Autodesk Fusion 360 part; units mm, degrees
(part 3 of 3)
  line L460 (365.2476, 258.4329) -> (365.2434, 258.3962)
  line L461 (365.4242, 258.127) -> (365.9464, 257.9803)
  line L462 (368.5391, 247.253) -> (369.0636, 246.6115)
  line L463 (368.5276, 247.6061) -> (368.8896, 247.9996)
  arc A277 (389.0677, 270.0365) -> (388.9102, 270.1312) centre (381.1421, 257.037) ccw
  line L464 (390.9137, 269.3965) -> (390.4979, 269.0483)
  line L465 (368.5391, 247.253) -> (368.5181, 247.2786)
  line L466 (359.931, 254.736) -> (359.9373, 254.7725)
  arc A278 (365.4068, 257.7213) -> (365.1921, 257.4738) centre (365.4421, 257.4738) ccw
  line L467 (386.2134, 242.1256) -> (385.951, 242.5914)
  line L468 (386.5528, 242.0274) -> (386.5219, 242.0153)
  line L469 (337.8939, 271.7181) -> (337.924, 271.7319)
  arc A279 (389.0905, 270.6345) -> (388.9718, 270.9399) centre (388.8551, 270.7188) ccw
  line L470 (365.9769, 261.9967) -> (365.9644, 261.9618)
  line L471 (365.6981, 261.0428) -> (365.5104, 260.2357)
  arc A280 (391.238, 269.3938) -> (390.9137, 269.3965) centre (391.0742, 269.2049) ccw
  line L472 (365.6509, 259.9116) -> (366.1529, 259.7063)
  line L473 (390.5886, 269.6398) -> (390.3522, 269.1604)
  line L474 (349.1921, 271.9615) -> (349.0339, 271.6922)
  line L475 (345.0126, 272.9687) -> (344.1728, 272.9927)
  line L476 (386.1921, 271.9615) -> (385.9174, 271.4938)
  line L477 (347.7954, 241.5055) -> (347.7633, 241.4971)
  line L478 (348.8153, 272.0785) -> (348.78, 271.7745)
  line L479 (383.0125, 241.1919) -> (383.8327, 241.3099)
  line L480 (382.3002, 241.324) -> (382.3711, 241.8617)
  line L481 (384.4579, 272.4399) -> (384.2384, 271.9439)
  line L482 (365.972, 252.7816) -> (366.5131, 252.8189)
  line L483 (365.5152, 253.8176) -> (365.5077, 253.8498)
  line L484 (367.9424, 265.9998) -> (367.4944, 265.3027)
  line L485 (347.7954, 241.5055) -> (348.608, 241.7191)
  line L486 (384.7859, 272.5711) -> (384.75, 272.5805)
  line L487 (339.6082, 272.3347) -> (339.6397, 272.3449)
  line L488 (367.5178, 264.9502) -> (367.9217, 264.5882)
  line L489 (382.0224, 241.1057) -> (382.0595, 241.1067)
  line L490 (349.2026, 242.1214) -> (349.0524, 242.3881)
  line L491 (383.0125, 241.1919) -> (382.9797, 241.1872)
  line L492 (345.0224, 241.1057) -> (345.0595, 241.1067)
  line L493 (349.5329, 272.0545) -> (349.4983, 272.0679)
  line L494 (339.9414, 272.2172) -> (340.0761, 271.9424)
  line L495 (345.3002, 241.324) -> (345.341, 241.6336)
  line L496 (367.3232, 264.5938) -> (367.8315, 264.428)
  line L497 (383.8116, 272.7672) -> (383.8444, 272.7625)
  line L498 (381.1941, 241.082) -> (382.0224, 241.1057)
  line L499 (347.7859, 272.5711) -> (347.75, 272.5805)
  line L500 (346.823, 272.7656) -> (345.9914, 272.8852)
  line L501 (341.3815, 272.7518) -> (340.5581, 272.5849)
  line L502 (346.0011, 241.1903) -> (345.9683, 241.1856)
  line L503 (367.0067, 264.4367) -> (367.0213, 264.4665)
  line L504 (381.1941, 241.082) -> (381.161, 241.0811)
  line L505 (367.0067, 264.4367) -> (366.6411, 263.6931)
  line L506 (341.6992, 272.5971) -> (341.8017, 272.3087)
  line L507 (367.9424, 265.9998) -> (367.9603, 266.0277)
  line L508 (365.7029, 253.0104) -> (365.7113, 252.9744)
  line L509 (384.0588, 272.5148) -> (384.0582, 271.9802)
  line L510 (366.092, 252.3937) -> (366.5651, 252.6426)
  line L511 (350.3158, 271.7496) -> (349.5329, 272.0545)
  line L512 (383.8116, 272.7672) -> (382.9914, 272.8852)
  line L513 (342.3537, 272.8921) -> (342.3169, 272.889)
  line L514 (365.6608, 254.1395) -> (366.1592, 254.3329)
  line L515 (340.3216, 272.3225) -> (340.3342, 272.0104)
  line L516 (365.9841, 252.0572) -> (366.2625, 251.2767)
  line L517 (346.0011, 241.1903) -> (346.8327, 241.3099)
  line L518 (382.9914, 272.8852) -> (382.9547, 272.8904)
  line L519 (367.4944, 265.3027) -> (367.4743, 265.2716)
  line L520 (380.9075, 241.2886) -> (380.8169, 241.8155)
  line L521 (340.5581, 272.5849) -> (340.5218, 272.5776)
  line L522 (365.5858, 254.5386) -> (366.1276, 254.514)
  line L523 (365.5152, 253.8176) -> (365.7029, 253.0104)
  line L524 (382.7042, 241.3645) -> (382.5542, 241.8777)
  line L525 (343.1909, 272.964) -> (342.3537, 272.8921)
  line L526 (383.8327, 241.3099) -> (383.8694, 241.3151)
  line L527 (345.287, 272.746) -> (345.3215, 272.4419)
  line L528 (385.8041, 272.0814) -> (385.7425, 271.5504)
  line L529 (365.9841, 252.0572) -> (365.9729, 252.0884)
  line L530 (385.5873, 272.3604) -> (384.7859, 272.5711)
  line L531 (384.0838, 241.5584) -> (384.0929, 242.1007)
  line L532 (368.5086, 266.4517) -> (368.8686, 266.046)
  line L533 (345.9914, 272.8852) -> (345.9547, 272.8904)
  line L534 (368.2747, 266.1198) -> (368.7607, 265.8972)
  line L535 (385.5873, 272.3604) -> (385.6193, 272.352)
  line L536 (344.1728, 272.9927) -> (344.1357, 272.9937)
  line L537 (348.829, 241.9946) -> (348.7987, 242.3055)
  arc A281 (388.1768, 271.3594) -> (387.8604, 271.2886) centre (388.0602, 271.1382) ccw
  arc A282 (369.3939, 267.5274) -> (369.071, 267.4717) centre (369.2646, 267.3134) ccw
  arc A283 (367.1471, 263.0319) -> (367.0757, 262.8626) centre (381.1421, 257.037) ccw
  arc A284 (382.9547, 272.8904) -> (382.6805, 272.7174) centre (382.9191, 272.643) ccw
  arc A285 (353.6743, 269.196) -> (353.4628, 269.3589) centre (344.1421, 257.037) ccw
  arc A286 (365.1921, 256.575) -> (365.4024, 256.3282) centre (365.4421, 256.575) ccw
  arc A287 (353.5982, 269.6333) -> (353.515, 269.9503) centre (353.3739, 269.7439) ccw
  arc A288 (367.4743, 265.2716) -> (367.5178, 264.9502) centre (367.6846, 265.1364) ccw
  line L538 (380.2007, 241.1092) -> (380.2376, 241.106)
  arc A289 (365.7113, 252.9744) -> (365.972, 252.7816) centre (365.9548, 253.031) ccw
  line L539 (380.4773, 272.7732) -> (380.5978, 272.2523)
  arc A290 (352.4494, 243.6553) -> (352.7749, 243.6177) centre (352.6338, 243.8241) ccw
  arc A291 (350.3595, 242.3414) -> (350.5132, 242.6269) centre (350.2688, 242.5744) ccw
  line L540 (366.7045, 263.3456) -> (367.1471, 263.0319)
  line L541 (381.1728, 272.9927) -> (381.1357, 272.9937)
  arc A292 (368.2747, 266.1198) -> (367.9603, 266.0277) centre (368.1706, 265.8925) ccw
  arc A293 (386.4983, 272.0679) -> (386.1921, 271.9615) centre (386.4076, 271.8349) ccw
  arc A294 (368.5021, 266.7759) -> (368.5086, 266.4517) centre (368.6956, 266.6176) ccw
  line L542 (382.2754, 272.7464) -> (382.3358, 272.2152)
  line L543 (366.5519, 262.9693) -> (367.0757, 262.8626)
  arc A295 (365.6608, 254.1395) -> (365.5077, 253.8498) centre (365.7512, 253.9064) ccw
  line L544 (382.6805, 272.7174) -> (382.5189, 272.1997)
  arc A296 (385.8041, 272.0814) -> (385.6193, 272.352) centre (385.5558, 272.1102) ccw
  arc A297 (367.9217, 264.5882) -> (367.8315, 264.428) centre (381.1421, 257.037) ccw
  arc A298 (369.9756, 267.3863) -> (369.8514, 267.2508) centre (381.1421, 257.037) ccw
  line L545 (366.2554, 262.7772) -> (366.2665, 262.8084)
  arc A299 (352.1007, 270.6291) -> (351.982, 270.9345) centre (351.8653, 270.7134) ccw
  arc A300 (366.5519, 262.9693) -> (366.2665, 262.8084) centre (366.5019, 262.7244) ccw
  line L546 (382.0011, 272.969) -> (382.0342, 272.968)
  arc A301 (384.0588, 272.5148) -> (383.8444, 272.7625) centre (383.8088, 272.5151) ccw
  line L547 (382.0011, 272.969) -> (381.1728, 272.9927)
  line L548 (345.6928, 241.3629) -> (345.6069, 241.6566)
  arc A302 (384.75, 272.5805) -> (384.4579, 272.4399) centre (384.6865, 272.3387) ccw
  arc A303 (382.2754, 272.7464) -> (382.0342, 272.968) centre (382.027, 272.7182) ccw
  arc A304 (350.8699, 242.7955) -> (351.189, 242.7211) centre (351.0723, 242.9422) ccw
  arc A305 (352.0143, 243.743) -> (352.2428, 243.881) centre (344.1421, 257.037) ccw
  arc A306 (365.3488, 254.7598) -> (365.5858, 254.5386) centre (365.5971, 254.7883) ccw
  arc A307 (366.092, 252.3937) -> (365.9729, 252.0884) centre (366.2084, 252.1724) ccw
  arc A308 (365.4314, 255.9231) -> (365.2463, 255.6528) centre (365.4947, 255.6813) ccw
  arc A309 (350.4476, 242.9323) -> (350.6903, 243.0433) centre (344.1421, 257.037) ccw
  arc A310 (381.1357, 272.9937) -> (380.883, 272.7906) centre (381.1286, 272.7438) ccw
  arc A311 (336.6123, 270.8712) -> (336.2895, 270.9273) centre (336.4186, 270.7132) ccw
  arc A312 (366.1276, 254.514) -> (366.1592, 254.3329) centre (381.1421, 257.037) ccw
  arc A313 (366.5131, 252.8189) -> (366.5651, 252.6426) centre (381.1421, 257.037) ccw
  arc A314 (369.6946, 268.1533) -> (369.6642, 267.8305) centre (369.8689, 267.974) ccw
  arc A315 (387.4886, 271.4519) -> (387.3359, 271.7418) centre (387.2452, 271.5088) ccw
  arc A316 (366.6248, 263.6599) -> (366.7045, 263.3456) centre (366.8491, 263.5496) ccw
  arc A317 (351.9941, 243.1459) -> (352.1143, 243.4471) centre (351.8774, 243.3671) ccw
  arc A318 (388.9406, 243.961) -> (389.0979, 244.0561) centre (381.1421, 257.037) ccw
  arc A319 (367.3232, 264.5938) -> (367.0213, 264.4665) centre (367.2457, 264.3561) ccw
  arc A320 (352.2261, 270.2033) -> (351.9975, 270.341) centre (344.1421, 257.037) ccw
  line L549 (349.542, 242.0232) -> (350.325, 242.328)
  arc A321 (335.5099, 270.4572) -> (335.4071, 270.1497) centre (335.639, 270.2431) ccw
  arc A322 (380.7815, 272.2578) -> (380.5978, 272.2523) centre (381.1421, 257.037) ccw
  arc A323 (350.4994, 271.4477) -> (350.3467, 271.7376) centre (350.256, 271.5046) ccw
  arc A324 (365.9379, 256.2419) -> (365.9486, 256.0584) centre (381.1421, 257.037) ccw
  line L550 (380.5015, 241.2944) -> (380.6332, 241.8205)
  line L551 (366.6411, 263.6931) -> (366.6248, 263.6599)
  line L552 (380.883, 272.7906) -> (380.7815, 272.2578)
  arc A325 (380.4773, 272.7732) -> (380.2124, 272.9659) centre (380.2338, 272.7168) ccw
  arc A326 (370.6663, 268.7982) -> (370.3392, 268.7797) centre (370.5134, 268.6004) ccw
  line L553 (380.1794, 272.9631) -> (380.2124, 272.9659)
  arc A327 (368.8686, 266.046) -> (368.7607, 265.8972) centre (381.1421, 257.037) ccw
  point P0 (365.1921, 257.6907)
  point P1 (365.1921, 256.362)
  point P2 (328.1921, 256.362)
  point P3 (328.1921, 257.7022)
  dimension "d364" = 30.45
  dimension "d365" = 0.25
  dimension "d366" = 0.25
  dimension "d367" = 0.25
  dimension "d368" = 0.25
  dimension "d369" = 7.5
  dimension "d370" = 30.9
  dimension "d371" = 0.25
  dimension "d372" = 0.25
  dimension "d373" = 0.25
  dimension "d374" = 0.25
  dimension "d375" = 7.5
  measures "d364" diameter of A58
  measures "d365" distance of L10.start P0
  measures "d366" distance of P1 L10.end
  measures "d367" radius of A278
  measures "d368" radius of A286
  measures "d369" diameter of A109
  measures "d370" diameter of A173
  measures "d371" distance of P3 L279.start
  measures "d372" distance of L272.start P2
  measures "d373" radius of A168
  measures "d374" radius of A219
  measures "d375" diameter of A169
extrude "Extrude1" add sketch "karaoke_machine_CNC" along normal blind 12.5 contours L0 L1 L10 L11 L12 A16 A17 L31 L32 L33 L34 L35 A34 A35 A36 L36 L37 L38 A37 L39 L40 L139 L140 L141 L142 L143 A74 A75 A76 A77 L144 L145 L146 L147 L148 L149 L150 L151 A78 A79 A80 L152 L153 L154 L155 L156 L157 A81 A82 A83 A84 makes body 1
extrude "Extrude2" add sketch "karaoke_machine_CNC" along normal blind 12.5 separate body contours L41 L42 L43 L44 A38 L45 L46 L47 L48 L49 L50 L51 L52 A39 A40 A41 makes body 2
extrude "Extrude3" add sketch "karaoke_machine_CNC" along normal blind 12.5 separate body contours A70 L127 L128 L129 A71 L130 L131 L132 A72 L133 L134 L135 A73 L136 L137 L138 makes body 3
extrude "Extrude4" add sketch "karaoke_machine_CNC" along normal blind 12.5 separate body contours L8 L9 L13 L14 L15 L16 L17 L18 L19 L20 L21 L22 L23 L24 A18 A19 A20 A21 A22 A23 A24 A25 A26 A27 A28 A29 A30 A31 A32 A33 L25 L26 L27 L28 L29 L30 makes body 4
extrude "Extrude5" add sketch "karaoke_machine_CNC" along normal blind 12.5 separate body contours A42 L53 A43 A44 L54 L55 A45 L56 L57 L58 L59 L60 L61 L62 L63 L64 makes body 5
extrude "Extrude6" add sketch "karaoke_machine_CNC" along normal blind 12.5 separate body contours A66 L115 L116 L117 A67 L118 L119 L120 A68 L121 L122 L123 A69 L124 L125 L126 makes body 6
extrude "Extrude7" add sketch "karaoke_machine_CNC" along normal blind 12.5 separate body contours L158 A85 A87 L159 A88 A89 L163 L165 L166 L168 L169 L170 A93 L172 L174 A94 A95 A96 L175 L176 L177 L178 L179 L180 L181 L182 L183 L184 L185 A97 A98 A99 L186 L187 L188 L189 L190 L191 L192 L193 L194 L195 A101 L196 A103 L197 A106 A112 L200 A114 A115 makes body 7
extrude "Extrude8" add sketch "karaoke_machine_CNC" along normal blind 12.5 separate body contours L5 L6 S2 S3 makes body 8
extrude "Extrude9" add sketch "karaoke_machine_CNC" along normal blind 12.5 separate body contours S0 L2 S1 L4 makes body 9
extrude "Extrude10" add sketch "karaoke_machine_CNC" along normal blind 12.5 separate body contours L90 L91 L92 L93 L94 L95 L96 L97 A51 A52 L98 L99 L100 L101 makes body 10
extrude "Extrude11" add sketch "karaoke_machine_CNC" along normal blind 12.5 separate body contours L65 L66 L67 L68 L69 L70 A46 L71 A47 L72 L73 L74 makes body 11
extrude "Extrude12" add sketch "karaoke_machine_CNC" along normal blind 12.5 separate body contours A49 L79 A50 L80 L81 L82 L83 L84 L85 L86 L87 L88 makes body 12
move_body "Move1" bodies 7 to x (1, 0, 0) y (0, -1, 0) z (0, 0, -1) at (0, 145.4868, -666.2204)
move_body "Move2" bodies 12 to x (0, 1, 0) y (-1, 0, 0) z (0, 0, 1) at (230.0825, 206.0825, 0)
move_body "Move3" bodies 11 to x (0, 1, 0) y (-1, 0, 0) z (0, 0, 1) at (226.7845, 202.7845, 0)
move_body "Move4" bodies 10 to x (0, 1, 0) y (-1, 0, 0) z (0, 0, 1) at (345.6956, 321.6956, 0)
move_body "Move5" bodies 11 to x (-1, 0, 0) y (0, -1, 0) z (0, 0, 1) at (24, 429.5689, 0)
move_body "Move6" bodies 2 to x (0, 1, 0) y (-1, 0, 0) z (0, 0, 1) at (402.4818, 378.4818, 0)
move_body "Move7" bodies 3 to x (0, 1, 0) y (-1, 0, 0) z (0, 0, 1) at (283.3048, 259.3048, 0)
move_body "Move8" bodies 4 to x (0, 0, -1) y (0, 1, 0) z (1, 0, 0) at (-189.1661, 0, 213.1661)
move_body "Move9" bodies 5 to x (0, 0, -1) y (0, 1, 0) z (1, 0, 0) at (-468.6693, 0, 492.6693)
move_body "Move10" bodies 6 to x (0, 0, -1) y (0, 1, 0) z (1, 0, 0) at (-255.1729, 0, 279.1729)
move_body "Move11" bodies 6 to x (1, 0, 0) y (0, 0.707107, 0.707107) z (0, -0.707107, 0.707107) at (0, 941.8633, 31.7011)
move_body "Align1" bodies 6 to x (1, 0, 0) y (0, 0.999999, 0.001039) z (0, -0.001039, 0.999999) at (0, -79.0434, 78.3441)
move_body "Align2" bodies 6 to x (1, 0, 0) y (0, 1, -0.000988) z (0, 0.000988, 1) at (1.8022, 4.2989, 3.0934)
move_body "Align3" bodies 6 to x (1, 0, 0) y (0, 1, 0.000988) z (0, -0.000988, 1) at (0, -0.7809, 0.4245)
move_body "Align4" bodies 6 to x (1, 0, 0) y (0, 1, 0) z (0, 0, 1) at (-1.2497, 0, 0)
move_body "Move12" bodies 6 to x (1, 0, 0) y (0, 1, 0) z (0, 0, 1) at (-452, 0, 0)
move_body "Align5" bodies 2 to x (1, 0, 0.000826) y (0, 1, -0.000004) z (-0.000826, 0.000004, 1) at (-387.3168, 109.4667, -427.7867)
move_body "Align6" bodies 4 to x (1, 0, 0) y (0, -0.999999, -0.001122) z (0, 0.001122, -0.999999) at (-396.0983, 185.4903, 525.4438)
move_body "Move13" bodies 4 to x (1, 0, 0) y (0, 1, 0) z (0, 0, 1) at (0, -110, -12.05)
move_body "Align7" bodies 3 to x (1, 0.000002, 0.00093) y (0, 0.999997, -0.002259) z (-0.00093, 0.002259, 0.999997) at (-451.5072, -260.7902, -458.4432)
move_body "Align8" bodies 5 to x (1, 0, 0) y (0, 1, -0.00004) z (0, 0.00004, 1) at (-200.9843, 404.2903, 82.7652)
move_body "Align9" bodies 7 to x (1, 0, 0) y (0, 0.999991, -0.004287) z (0, 0.004287, 0.999991) at (-451.9991, 19.7942, 983.8967)
move_body "Align10" bodies 12 to x (1, 0, 0) y (0, -0.999999, -0.001109) z (0, 0.001109, -0.999999) at (19.702, 432.115, 594.5361)
move_body "Move14" bodies 12 to x (1, 0, 0) y (0, 1, 0) z (0, 0, 1) at (0, 12.05, 0)
move_body "Align11" bodies 10 to x (1, 0, 0) y (0, 1, 0.000269) z (0, -0.000269, 1) at (-2.5, -66.0667, 282.7746)
move_body "Align12" bodies 11 to x (1, 0, 0) y (0, 0.99997, -0.007739) z (0, 0.007739, 0.99997) at (-486.4991, 45.7749, 197.5774)
sketch "useless dowel sketch" plane through (-439.4991, 0, 0) normal (1, 0, 0) x (0, 0, -1)
  circle A0 centre (-299.0465, 453.4309) radius 7.88
  arc A1 (-409.7254, 271.7142) -> (-412.2122, 274.2273) centre (-409.7123, 274.2142) ccw
  line L0 (-409.7254, 271.7142) -> (-409.7572, 264.2062)
  arc A2 (-412.2668, 261.7157) -> (-409.7572, 264.2062) centre (-409.7668, 261.7062) ccw
  line L1 (-412.2668, 261.7157) -> (-457.4665, 261.8774)
  arc A3 (-459.9573, 264.3866) -> (-457.4665, 261.8774) centre (-459.9665, 261.8867) ccw
  line L2 (-459.9573, 264.3866) -> (-459.9276, 272.0866)
  arc A4 (-457.4183, 274.5772) -> (-459.9276, 272.0866) centre (-459.9183, 274.5866) ccw
  line L3 (-457.4183, 274.5772) -> (-412.2122, 274.2273)
  arc A5 (-427.6008, 301.0556) -> (-431.5836, 305.0727) centre (-431.6008, 301.0727) ccw
  line L4 (-427.6008, 301.0556) -> (-427.6737, 284.0557)
  arc A6 (-431.6908, 280.0729) -> (-427.6737, 284.0557) centre (-431.6736, 284.0729) ccw
  line L5 (-431.6908, 280.0729) -> (-437.6907, 280.0986)
  arc A7 (-441.6735, 284.1158) -> (-437.6907, 280.0986) centre (-437.6736, 284.0986) ccw
  line L6 (-441.6735, 284.1158) -> (-441.6007, 301.1156)
  arc A8 (-437.5836, 305.0984) -> (-441.6007, 301.1156) centre (-437.6007, 301.0984) ccw
  line L7 (-437.5836, 305.0984) -> (-431.5836, 305.0727)
  circle A9 centre (-380.0945, 179.9508) radius 4
  circle A10 centre (-385.3516, 119.9728) radius 4
  circle A11 centre (-450.4796, 90.2517) radius 4
  circle A12 centre (-447.1439, 291.0393) radius 4
  circle A13 centre (-399.3656, 350.035) radius 4
  line L8 (-75.851, -1.3491) -> (-75.6774, 40.6676)
  arc A14 (-75.6774, 40.6676) -> (-83.4677, 50.4617) centre (-85.6774, 40.7089) ccw
  line L9 (-83.4677, 50.4617) -> (-298.823, 99.2538)
  arc A15 (-300.381, 101.2116) -> (-298.823, 99.2538) centre (-298.3811, 101.2043) ccw
  line L10 (-300.381, 101.2116) -> (-300.3608, 106.7978)
  line L11 (-300.3608, 106.7978) -> (-310.3958, 106.8942)
  arc A16 (-312.8658, 109.424) -> (-310.3958, 106.8942) centre (-312.8956, 106.9242) ccw
  line L12 (-312.8658, 109.424) -> (-312.6888, 124.6362)
  arc A17 (-310.1596, 127.1061) -> (-312.6888, 124.6362) centre (-312.6594, 127.136) ccw
  line L13 (-310.1596, 127.1061) -> (-300.1102, 126.9963)
  line L14 (-300.1102, 126.9963) -> (-299.8561, 217.1017)
  line L15 (-299.8561, 217.1017) -> (-309.9059, 217.1756)
  arc A18 (-312.3918, 219.668) -> (-309.9059, 217.1756) centre (-312.4059, 217.1681) ccw
  line L16 (-312.3918, 219.668) -> (-312.4322, 234.7111)
  arc A19 (-309.944, 237.3679) -> (-312.4322, 234.7111) centre (-312.4391, 237.2111) ccw
  line L17 (-309.944, 237.3679) -> (-299.7403, 237.3013)
  line L18 (-299.7403, 237.3013) -> (-299.6828, 247.3323)
  arc A20 (-297.9827, 251.0601) -> (-299.6828, 247.3323) centre (-294.6829, 247.3036) ccw
  line L19 (-297.9827, 251.0601) -> (-81.4515, 441.2735)
  arc A21 (-81.4515, 441.2735) -> (-80.9389, 455.816) centre (-88.0513, 448.7864) ccw
  line L20 (-80.9389, 455.816) -> (-100.8396, 475.951)
  line L21 (-100.8396, 475.951) -> (-107.9384, 468.8386)
  arc A22 (-111.4739, 468.8352) -> (-107.9384, 468.8386) centre (-109.7044, 467.0691) ccw
  line L22 (-111.4739, 468.8352) -> (-122.2331, 479.572)
  arc A23 (-122.2365, 483.1075) -> (-122.2331, 479.572) centre (-124.0025, 481.3381) ccw
  line L23 (-122.2365, 483.1075) -> (-115.1369, 490.2208)
  line L24 (-115.1369, 490.2208) -> (-123.7067, 498.8673)
  line L25 (-123.7067, 498.8673) -> (-178.5271, 499.0981)
  line L26 (-178.5271, 499.0981) -> (-178.5681, 489.536)
  arc A24 (-181.2287, 487.0519) -> (-178.5681, 489.536) centre (-178.7287, 487.0412) ccw
  line L27 (-181.2287, 487.0519) -> (-196.2761, 487.1163)
  arc A25 (-198.7679, 489.6264) -> (-196.2761, 487.1163) centre (-198.7761, 487.1264) ccw
  line L28 (-198.7679, 489.6264) -> (-198.727, 499.1844)
  line L29 (-198.727, 499.1844) -> (-373.7298, 499.9308)
  line L30 (-373.7298, 499.9308) -> (-564.202, 334.7144)
  arc A26 (-564.202, 334.7144) -> (-574.5443, 312.1828) centre (-544.5445, 312.052) ccw
  line L31 (-574.5443, 312.1828) -> (-575.0343, 199.8165)
  line L32 (-575.0343, 199.8165) -> (-564.9844, 199.7675)
  arc A27 (-562.4966, 197.2555) -> (-564.9844, 199.7675) centre (-562.4844, 199.7554) ccw
  line L33 (-562.4966, 197.2555) -> (-562.8415, 182.2067)
  arc A28 (-565.35, 179.569) -> (-562.8415, 182.2067) centre (-562.8538, 179.7068) ccw
  line L34 (-565.35, 179.569) -> (-575.1322, 179.6167)
  line L35 (-575.1322, 179.6167) -> (-575.7522, 25.79)
  line L36 (-575.7522, 25.79) -> (-550.8677, 0.6896)
  line L37 (-550.8677, 0.6896) -> (-230.6816, -0.7538)
  line L38 (-230.6816, -0.7538) -> (-230.6485, 9.2961)
  arc A29 (-228.1395, 11.787) -> (-230.6485, 9.2961) centre (-230.6394, 11.7961) ccw
  line L39 (-228.1395, 11.787) -> (-212.9437, 11.7809)
  arc A30 (-210.4487, 9.2759) -> (-212.9437, 11.7809) centre (-210.4437, 11.7759) ccw
  line L40 (-210.4487, 9.2759) -> (-210.4818, -0.8315)
  line L41 (-210.4818, -0.8315) -> (-75.851, -1.3491)
  circle A31 centre (-475, 495) radius 4
  dimension "d400" = 8
  measures "d400" diameter of A31
extrude "Extrude13" add sketch "useless dowel sketch" along normal blind 480 separate body contours A31 makes body 13
copy_body "CopyPasteBodies1" bodies 13 makes body 14
move_body "Move15" bodies 14 to x (1, 0, 0) y (0, 1, 0) z (0, 0, 1) at (0, 0, 25)
copy_body "CopyPasteBodies2" bodies 13 makes body 15
move_body "Move16" bodies 15 to x (1, 0, 0) y (0, 1, 0) z (0, 0, 1) at (0, 0, 50)
copy_body "CopyPasteBodies3" bodies 13 makes body 16
move_body "Move17" bodies 16 to x (1, 0, 0) y (0, 1, 0) z (0, 0, 1) at (0, 0, 100)
copy_body "CopyPasteBodies4" bodies 13 makes body 17
move_body "Move18" bodies 17 to x (1, 0, 0) y (0, 1, 0) z (0, 0, 1) at (0, 0, 150)
copy_body "CopyPasteBodies5" bodies 13 makes body 18
move_body "Move19" bodies 18 to x (1, 0, 0) y (0, 1, 0) z (0, 0, 1) at (0, 0, 200)
move_body "Align13" bodies 13 to x (1, 0, 0) y (0, 1, 0) z (0, 0, 1) at (-28.0009, -41.175, -174.875)
move_body "Align14" bodies 14 to x (1, 0, 0) y (0, 1, 0) z (0, 0, 1) at (-28.0009, -145, -100)
move_body "Align15" bodies 15 to x (1, 0, 0) y (0, 1, 0) z (0, 0, 1) at (-28.0009, -204.2, -77.475)
move_body "Align16" bodies 16 to x (1, 0, 0) y (0, 1, 0) z (0, 0, 1) at (-28.0009, -315, -195)
move_body "Align17" bodies 17 to x (1, 0, 0) y (0, 1, 0) z (0, 0, 1) at (-28.0009, -375, -240)
move_body "Align18" bodies 18 to x (1, 0, 0) y (0, 1, 0) z (0, 0, 1) at (-28.0009, -405, -225)
move_body "Align19" bodies 9 to x (1, 0, 0) y (0, 1, 0) z (0, 0, 1) at (0, -155.2652, 493.7005)
move_body "Move20" bodies 9 to x (1, 0, 0) y (0, 1, 0) z (0, 0, 1) at (-350, 0, 0)
move_body "Align20" bodies 8 to x (1, 0, 0) y (0, 1, 0) z (0, 0, 1) at (0, -192.4606, 423.537)
move_body "Move21" bodies 8 to x (1, 0, 0) y (0, 1, 0) z (0, 0, 1) at (-125, 0, 0)
copy_body "CopyPasteBodies6" bodies 1 13 18 5 6 9 10 12 4 14 15 7 16 17 3 8 11 2 makes body 19 makes body 20 makes body 21 makes body 22 makes body 23 makes body 24 makes body 25 makes body 26 makes body 27 makes body 28 makes body 29 makes body 30 makes body 31 makes body 32 makes body 33 makes body 34 makes body 35 makes body 36
move_body "Move22" bodies 19 to x (0, -1, 0) y (1, 0, 0) z (0, 0, 1) at (0, 0, 0)
move_body "Move23" bodies 30 to x (0, -1, 0) y (1, 0, 0) z (0, 0, 1) at (3.1991, -451.9293, 551.0525)
move_body "Move24" bodies 19 to x (1, 0, 0) y (0, 1, 0) z (0, 0, 1) at (182.8554, 0, 35.2992)
move_body "Move25" bodies 30 to x (1, 0, 0) y (0, 1, 0) z (0, 0, 1) at (186.8271, 0, 68.7985)
sketch "Sketch5" plane through (0, 0.023, 575.4507) normal (0, 0.00004, 1) x (1, 0, 0)
  line L0 (-452.4982, 178.7955) -> (-442.4982, 178.7955)
  arc A0 (-439.9986, 176.2951) -> (-442.4982, 178.7955) centre (-439.9982, 178.7951) ccw
  line L1 (-439.9986, 176.2951) -> (-439.9986, 168.8065)
  line L2 (-439.9986, 168.8065) -> (0.0565, 168.8065)
  line L3 (0.0565, 168.8065) -> (0.0565, 176.3331)
  arc A1 (2.5564, 178.8332) -> (0.0565, 176.3331) centre (0.0564, 178.8331) ccw
  line L4 (2.5564, 178.8332) -> (12.5, 178.8332)
  line L5 (12.5, 178.8332) -> (12.5, 198.8332)
  line L6 (12.5, 198.8332) -> (2.5, 198.8332)
  arc A2 (-0.0005, 201.3331) -> (2.5, 198.8332) centre (0, 198.8331) ccw
  line L7 (-0.0005, 201.3331) -> (-0.0005, 208.8065)
  line L8 (-0.0005, 208.8065) -> (-440.0005, 208.8065)
  line L9 (-440.0005, 208.8065) -> (-440.0005, 201.2951)
  arc A3 (-442.5008, 198.7955) -> (-440.0005, 201.2951) centre (-440.0008, 198.7951) ccw
  line L10 (-442.5008, 198.7955) -> (-452.4982, 198.7955)
  line L11 (-452.4982, 198.7955) -> (-452.4982, 178.7955)
move_body "Move26" bodies 22 to x (1, 0, 0) y (0, 0, -1) z (0, 1, 0) at (1266.3396, -394.0977, 432.5484)
move_body "Move27" bodies 23 to x (1, 0, 0) y (0, 1, 0) z (0, 0, 1) at (2136.0119, 0, 162.9247)
move_body "Align21" bodies 23 to x (1, 0, 0) y (0, 0.707869, 0.706343) z (0, -0.706343, 0.707869) at (-870.1722, 30.7907, -289.2908)
move_body "Move28" bodies 22 to x (1, 0, 0) y (0, 1, 0) z (0, 0, 1) at (0, 0, -75)
move_body "Move29" bodies 36 to x (1, 0, 0) y (0, 1, 0) z (0, 0, 1) at (1733.338, 0, 122.4679)
move_body "Move30" bodies 24 to x (0, -1, 0) y (1, 0, 0) z (0, 0, 1) at (792.1717, -320, 39.6421)
move_body "Move31" bodies 34 to x (0, -1, 0) y (1, 0, 0) z (0, 0, 1) at (1007.8683, -95, -100.3325)
move_body "Move32" bodies 27 to x (1, 0, 0) y (0, 0, -1) z (0, 1, 0) at (514.7679, -202.4713, 19.8925)
move_body "Align22" bodies 33 to x (1, 0, 0) y (0, 0.999997, 0.002259) z (0, -0.002259, 0.999997) at (0, -12.0508, -0.0278)
move_body "Align23" bodies 24 to x (1, 0, 0) y (0, 1, 0) z (0, 0, 1) at (0, -30, 0)
move_body "Align24" bodies 34 to x (1, 0, 0) y (0, 1, 0) z (0, 0, 1) at (-215.6966, -30, 139.9745)
move_body "Move33" bodies 24 to x (1, 0, 0) y (0, 1, 0) z (0, 0, 1) at (1.2371, 0, 220.7292)
move_body "Align25" bodies 23 to x (1, 0, 0) y (0, 1, 0.00004) z (0, -0.00004, 1) at (0, -181.3357, -0.0073)
move_body "Align26" bodies 36 to x (1, 0, 0) y (0, 1, 0.000004) z (0, -0.000004, 1) at (-466.9981, -500.4496, -68.5338)
move_body "Align27" bodies 22 to x (1, 0, 0) y (0, 1, 0.00004) z (0, -0.00004, 1) at (0, -181.3387, 74.9927)
move_body "Move34" bodies 22 to x (1, 0, 0) y (0, 1, 0) z (0, 0, 1) at (0, 0, -75)
move_body "Move35" bodies 23 to x (1, 0, 0) y (0, 1, 0) z (0, 0, 1) at (0, 0, 75)
move_body "Align28" bodies 27 to x (1, 0, 0) y (0, 0.999999, -0.001122) z (0, 0.001122, 0.999999) at (751.5017, -110.1938, 321.3745)
move_body "Align29" bodies 33 to x (1, 0, 0) y (0, 1, 0) z (0, 0, 1) at (1266.3375, 0, -51.0962)
move_body "Align30" bodies 25 to x (1, 0, 0) y (0, 1, -0.000269) z (0, 0.000269, 1) at (0, -268.205, 0.0721)
move_body "Align31" bodies 26 to x (1, 0, 0) y (0, 0.999999, -0.001109) z (0, 0.001109, 0.999999) at (0, -238.7415, 0.2645)
move_body "Align32" bodies 35 to x (1, 0, 0) y (0, 0.99997, 0.007739) z (0, -0.007739, 0.99997) at (0, -271.0288, -2.1107)
sketch "Sketch6" plane through (0, 0, 0) normal (0, 1, 0) x (1, 0, 0)
  line L0 (1500, -100) -> (2100, -100)
  line L1 (2100, -100) -> (2100, -700)
  line L2 (2100, -700) -> (1500, -700)
  line L3 (1500, -700) -> (1500, -100)
  dimension "d405" = 600
  dimension "d406" = 600
  measures "d405" distance of L0.start L0.end
  measures "d406" distance of L0.start L2.end
move_body "Move36" bodies 19 to x (1, 0, 0) y (0, 1, 0) z (0, 0, 1) at (1337.7026, 0, 466.0774)
move_body "Move37" bodies 24 to x (1, 0, 0) y (0, 1, 0) z (0, 0, 1) at (880.7047, 0, -12.1059)
move_body "Move38" bodies 34 to x (1, 0, 0) y (0, 1, 0) z (0, 0, 1) at (817.1487, 0, 145.2709)
move_body "Move39" bodies 30 to x (-1, 0, 0) y (0, 1, 0) z (0, 0, -1) at (803.9005, 0, 1692.4912)
sketch "Sketch7" plane through (0, 0, 0) normal (0, 1, 0) x (1, 0, 0)
  line L0 (2200, -100) -> (2800, -100)
  line L1 (2800, -100) -> (2800, -1100)
  line L2 (2800, -1100) -> (2200, -1100)
  line L3 (2200, -1100) -> (2200, -100)
  dimension "d407" = 600
  dimension "d408" = 1000
  measures "d407" distance of L0.start L0.end
  measures "d408" distance of L0.start L2.end
move_body "Move40" bodies 30 to x (-1, 0, 0) y (0, 1, 0) z (0, 0, -1) at (2841.6045, 0, 1565.1355)
move_body "Move41" bodies 33 to x (1, 0, 0) y (0, 1, 0) z (0, 0, 1) at (1416.1072, 0, -12.7119)
move_body "Move42" bodies 23 to x (1, 0, 0) y (0, 1, 0) z (0, 0, 1) at (1418.6496, 0, -104.2377)
move_body "Move43" bodies 22 to x (1, 0, 0) y (0, 1, 0) z (0, 0, 1) at (1438.9887, 0, 124.5768)
move_body "Move44" bodies 27 to x (1, 0, 0) y (0, 1, 0) z (0, 0, 1) at (1421.192, 0, 233.8992)
move_body "Move45" bodies 36 to x (1, 0, 0) y (0, 1, 0) z (0, 0, 1) at (706.7824, 0, 244.0687)
move_body "Move46" bodies 35 to x (1, 0, 0) y (0, 1, 0) z (0, 0, 1) at (2860.1806, 0, 294.9164)
move_body "Move47" bodies 26 to x (1, 0, 0) y (0, 1, 0) z (0, 0, 1) at (2356.7888, 0, 211.0178)
move_body "Move48" bodies 25 to x (1, 0, 0) y (0, 1, 0) z (0, 0, 1) at (2438.1451, 0, 238.984)
move_body "Move49" bodies 36 to x (1, 0, 0) y (0, 1, 0) z (0, 0, 1) at (714.5058, 0, 29.7711)
move_body "Move50" bodies 26 to x (1, 0, 0) y (0, 1, 0) z (0, 0, 1) at (-49.7194, 0, -46.6045)
move_body "Move51" bodies 25 to x (1, 0, 0) y (0, 1, 0) z (0, 0, 1) at (-57.0319, 0, -74.0968)
move_body "Move52" bodies 35 to x (1, 0, 0) y (0, 1, 0) z (0, 0, 1) at (114.7848, 0, -129.7428)
move_body "Move53" bodies 24 to x (0.906308, 0, 0.422618) y (0, 1, 0) z (-0.422618, 0, 0.906308) at (1092.2758, 0, -668.4104)
move_body "Move54" bodies 34 to x (1, 0, 0) y (0, 1, 0) z (0, 0, 1) at (957.3304, 0, 401.2365)
move_body "Move55" bodies 19 to x (1, 0, 0) y (0, 1, 0) z (0, 0, 1) at (35.2516, 0, -445.6807)
move_body "Move56" bodies 19 20 21 27 34 29 25 24 26 30 31 33 28 32 23 22 36 35 to x (1, 0, 0) y (0, 0, -1) z (0, 1, 0) at (0, -142.6958, 118.6958)
hidden bodies 20 28 29 31 32
equation "motor_h = 38.9 mm"
equation "motor_w = 42.35 mm"
equation "screw_diameter_full = 2.89 mm"
equation "screw_diameter_hole = 2.58 mm"
equation "distance_btw_holes_edges = 28.7 mm"
equation "device_height = 500 mm"
equation "dowel_diameter = 8 mm"
equation "bearing_outer_diameter = 16.01 mm"
equation "USED_bearing_outer_diameter = bearing_outer_diameter - 0.25 mm"
equation "motor_head_diameter = 17.07 mm"
equation "motor_head_hole = motor_head_diameter + 0.12 mm"
equation "motor_head_length = 17.1 mm"
equation "motor_head_gears_length = 8.2 mm"
equation "MOTOR_GEAR_portrusion = 0.6 mm"
equation "MOTOR_GEAR_out_w = 0.9 mm"
equation "MOTOR_GEAR_in_w = 1.3 mm"
equation "motor_head_gears_diameter_full = 12.48 mm"
equation "number_of_motor_gears = 20"
equation "wood_width = 12.5 mm"
equation "rod_to_band_distance = 1.5 mm"
equation "gearwheel_diameter_1 = 30 mm"
equation "gearwheel_diameter_2 = gearwheel_diameter_1 + 0.25 mm"
equation "gearwheel_diameter_3 = gearwheel_diameter_1 + 0.45 mm"
equation "math_mhD_mgD = ( motor_head_diameter - motor_head_gears_diameter_full ) / 2"
equation "math_mh_dist_var = ( motor_head_hole / 2 ) - math_mhD_mgD"
equation "dowel_hole_to_motor_hold_distance = math_mh_dist_var + ( gearwheel_diameter_1 / 2 )"
equation "A3_w = 420 mm"
equation "device_positionary_width = 500 mm"
equation "device_inner_width = A3_w + 20 mm"
equation "d40 = motor_head_hole"
equation "d54 = screw_diameter_full"
equation "d55 = screw_diameter_full"
equation "d56 = screw_diameter_full"
equation "d57 = screw_diameter_full"
equation "d58 = dowel_hole_to_motor_hold_distance"
equation "d60 = dowel_diameter"
equation "d86 = USED_bearing_outer_diameter"
equation "d87 = dowel_diameter"
equation "d88 = dowel_diameter"
equation "d89 = dowel_diameter"
equation "d90 = dowel_diameter"
equation "d91 = dowel_diameter"
equation "d92 = dowel_diameter"
equation "d96 = dowel_diameter"
equation "d97 = dowel_diameter"
equation "d98 = dowel_diameter"
equation "d99 = wood_width + 0.05 mm"
equation "d103 = wood_width"
equation "d105 = wood_width"
equation "d116 = device_inner_width"
equation "d117 = device_inner_width"
equation "d118 = wood_width"
equation "d121 = wood_width"
equation "d129 = wood_width + 0.05 mm"
equation "d134 = wood_width"
equation "d137 = device_inner_width"
equation "d138 = wood_width"
equation "d144 = wood_width"
equation "d146 = device_inner_width"
equation "d147 = wood_width"
equation "d164 = dowel_diameter"
equation "d166 = motor_w"
equation "d167 = motor_w"
equation "d216 = dowel_diameter"
equation "d218 = wood_width + 0.2 mm"
equation "d223 = wood_width + 0.2 mm"
equation "d229 = wood_width"
equation "d231 = device_inner_width"
equation "d232 = wood_width"
equation "d238 = wood_width"
equation "d240 = device_inner_width"
equation "d241 = wood_width"
equation "d247 = wood_width + 0.05 mm"
equation "d252 = wood_width + 0.05 mm"
equation "d262 = wood_width + 0.05 mm"
equation "d274 = dowel_diameter"
equation "d275 = USED_bearing_outer_diameter"
equation "d276 = dowel_diameter"
equation "d277 = dowel_diameter"
equation "d278 = dowel_diameter"
equation "d279 = wood_width + 0.05 mm"
equation "d285 = wood_width + 0.05 mm"
equation "d291 = dowel_diameter"
equation "d293 = wood_width + 0.2 mm"
equation "d304 = wood_width + 0.05 mm"
equation "d309 = wood_width + 0.05 mm"
equation "d315 = wood_width + 0.05 mm"
equation "gearwheel_diameter_4 = gearwheel_diameter_1 + 0.9 mm"
equation "d364 = gearwheel_diameter_3"
equation "d369 = dowel_diameter - 0.5 mm"
equation "d370 = gearwheel_diameter_4"
equation "d375 = dowel_diameter - 0.5 mm"
equation "d376 = wood_width"
equation "d378 = wood_width"
equation "d380 = wood_width"
equation "d382 = wood_width"
equation "d384 = wood_width"
equation "d386 = wood_width"
equation "d388 = wood_width"
equation "d390 = wood_width"
equation "d392 = wood_width"
equation "d394 = wood_width"
equation "d396 = wood_width"
equation "d398 = wood_width"
equation "d400 = dowel_diameter"
